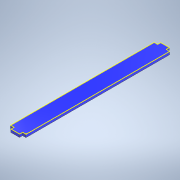
# Autodesk Inventor part: chassis_1_3
Saved by Autodesk Inventor 2022 (Build 260153000, 153)
## iProperties
Created: 2023-03-24
Part Number: chassis_1_3
Material: 一般
Document SubType Name: Modeling
Designer: Johnny Jou
Density: 1 g/cm^3
Appearance: 預設
Author: Johnny Jou
Autodesk Inventor part; units mm, degrees
ref_plane "YZ Plane" through (0, 0, 0) normal (1, 0, 0) x (0, 1, 0)
ref_plane "XZ Plane" through (0, 0, 0) normal (0, 1, 0) x (-1, 0, 0)
ref_plane "XY Plane" through (0, 0, 0) normal (0, 0, 1) x (1, 0, 0)
sketch "草圖1" plane through (0, 0, 0) normal (0, 1, 0) x (-1, 0, 0)
  line L0 (0, 0) -> (0, -140)
  line L1 (15, -140) -> (15, 0)
  line L2 (3.35, 0) -> (3.35, 3)
  line L3 (3.35, 3) -> (11.65, 3)
  line L4 (11.65, 3) -> (11.65, 0)
  line L5 (3.35, -140) -> (3.35, -143)
  line L6 (3.35, -143) -> (11.65, -143)
  line L7 (11.65, -143) -> (11.65, -140)
  line L8 (0, -140) -> (3.35, -140)
  line L9 (11.65, -140) -> (15, -140)
  line L10 (15, 0) -> (11.65, 0)
  line L11 (3.35, 0) -> (0, 0)
  dimension "d0" = 3
  dimension "d1" = 8.3
  dimension "d2" = 15
  dimension "d3" = 3.35
  dimension "d4" = 3
  dimension "d5" = 8.3
  dimension "d6" = 3.35
  dimension "d7" = 140
  dimension "d8" = 140
  constraints: 24 end point, 7 parallel, 2 horizontal, 2 perpendicular, 1 coincident, 1 horizontal alignment
  measures "d0" distance of L6.end L7.end
  measures "d1" distance of L5.end L6.end
  measures "d2" distance between parallel lines of L0 L1
  measures "d3" distance between parallel lines of L1 L7
  measures "d4" distance of L3.end L4.end
  measures "d5" distance of L2.end L3.end
  measures "d6" distance between parallel lines of L1 L4
  measures "d7" distance of L1.start L1.end
  measures "d8" distance of L0.start L0.end
extrude "擠出1" add sketch "草圖1" along normal blind 3
sketch "草圖2" plane through (0, 3, 0) normal (0, 1, 0) x (1, 0, 0)
  line L0 (0, 0) -> (0, 140) projected
  line L1 (0, 140) -> (-3.35, 140) projected
  line L2 (-3.35, 140) -> (-3.35, 143) projected
  line L3 (-3.35, 143) -> (-11.65, 143) projected
  line L4 (-11.65, 143) -> (-11.65, 140) projected
  line L5 (-11.65, 140) -> (-15, 140) projected
  line L6 (-15, 140) -> (-15, 0) projected
  line L7 (-15, 0) -> (-11.65, 0) projected
  line L8 (-11.65, 0) -> (-11.65, -3) projected
  line L9 (-11.65, -3) -> (-3.35, -3) projected
  line L10 (-3.35, -3) -> (-3.35, 0) projected
  line L11 (-3.35, 0) -> (0, 0) projected
equation "\"d3\" = -0.5 * d1 + 0.5 * d2"
equation "\"d6\" = d3"
